Autodesk Inventor part; units mm, degrees
(part 3 of 3)
  line L372 (-9.4727, -16.9965) -> (-8.9155, -16.4393) projected
  line L373 (-10.552, -17.5763) -> (-10.5765, -17.5519) projected
  line L374 (-10.5765, -17.5519) -> (-10.9223, -17.8977) projected
  line L375 (-13.8024, -11.0005) -> (-15.4197, -12.6178) projected
  line L376 (-15.4197, -12.6178) -> (-15.1472, -12.8903) projected
  line L377 (-15.1472, -12.8903) -> (-13.5299, -11.273) projected
  line L378 (-13.5299, -11.273) -> (-13.8024, -11.0005) projected
  line L379 (-16.2092, -10.5708) -> (-15.3551, -11.4249) projected
  line L380 (-15.5559, -9.4461) -> (-15.8529, -9.743) projected
  line L381 (-15.8529, -9.743) -> (-15.8371, -9.7587) projected
  line L382 (-15.1472, -11.2171) -> (-16.2668, -10.0975) projected
  line L383 (-16.2668, -10.0975) -> (-16.4152, -10.246) projected
  line L384 (-16.0397, -8.7632) -> (-18.2911, -11.0145) projected
  line L385 (-18.2911, -11.0145) -> (-18.0186, -11.2869) projected
  line L386 (-18.0186, -11.2869) -> (-15.7673, -9.0356) projected
  line L387 (-15.7673, -9.0356) -> (-16.0397, -8.7632) projected
  circle A0 centre (-12.4372, -30.0261) radius 2.75 projected
  circle A1 centre (12.4372, -30.0261) radius 2.75 projected
  circle A2 centre (30.0261, -12.4372) radius 2.75 projected
  circle A3 centre (30.0261, 12.4372) radius 2.75 projected
  circle A4 centre (12.4372, 30.0261) radius 2.75 projected
  circle A5 centre (-22.981, 22.981) radius 2.75 projected
  circle A6 centre (-32.5, 0) radius 2.75 projected
  circle A7 centre (0, 32.5) radius 2.75 projected
  circle A8 centre (-30.0261, -12.4372) radius 2.75 projected
  circle A9 centre (-30.0261, 12.4372) radius 2.75 projected
  circle A10 centre (-12.4372, 30.0261) radius 2.75 projected
  circle A11 centre (22.981, 22.981) radius 2.75 projected
  circle A12 centre (32.5, 0) radius 2.75 projected
  circle A13 centre (22.981, -22.981) radius 2.75 projected
  circle A14 centre (0, -32.5) radius 2.75 projected
  circle A15 centre (-22.981, -22.981) radius 2.75 projected
  circle A16 centre (8, 0) radius 2.1 projected
  circle A17 centre (-8, 0) radius 2.1 projected
  circle A18 centre (0, -8) radius 2.1 projected
  circle A19 centre (0, 8) radius 2.1 projected
  circle A20 centre (0, 0) radius 40 projected
  constraints: 429 other
